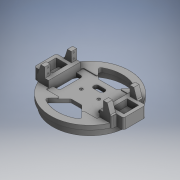
# Autodesk Inventor part: Swivel Top
Saved by Autodesk Inventor 2020.5 (Build 245400000, 400)
## iProperties
Created: 2023-04-01
Part Number: Swivel Top
Material: Generic
Document SubType Name: Modeling
Designer: Wes
Density: 1 g/cm^3
Appearance: Default
Author: Wes
Autodesk Inventor part; units mm, degrees
ref_plane "YZ Plane" through (0, 0, 0) normal (1, 0, 0) x (0, 1, 0)
ref_plane "XZ Plane" through (0, 0, 0) normal (0, 1, 0) x (-1, 0, 0)
ref_plane "XY Plane" through (0, 0, 0) normal (0, 0, 1) x (1, 0, 0)
sketch "Sketch1" plane through (0, 0, 0) normal (0, 0, 1) x (1, 0, 0)
  circle A0 centre (0, 0) radius 74
  dimension "d0" = 148
  constraints: 1 centre point, 1 coincident
  measures "d0" diameter of A0
extrude "Extrusion1" add sketch "Sketch1" along normal blind 8
sketch "Sketch2" plane through (0, 0, 8) normal (0, 0, 1) x (1, 0, 0)
  line L0 (0, 0) -> (0, -55) construction
  line L1 (0, 0) -> (0, 55) construction
  line L2 (0, -55) -> (0, -48) construction
  line L3 (0, -48) -> (-30, -48) construction
  line L4 (0, -48) -> (30, -48) construction
  line L5 (-30, -48) -> (30, -48)
  line L6 (30, -48) -> (30, -71)
  line L7 (30, -71) -> (-30, -71)
  line L8 (-30, -71) -> (-30, -48)
  line L9 (0, -71) -> (0, -84) construction
  line L10 (0, -84) -> (-21, -84) construction
  line L11 (0, -84) -> (21, -84) construction
  line L12 (-21, -84) -> (21, -84)
  line L13 (21, -84) -> (21, -71)
  line L14 (21, -71) -> (-21, -71)
  line L15 (-21, -71) -> (-21, -84)
  dimension "d3" = 55
  dimension "d5" = 7
  dimension "d7" = 30
  dimension "d8" = 60
  dimension "d9" = 23
  dimension "d10" = 13
  dimension "d11" = 21
  dimension "d13" = 42
  dimension "d14" = 13
  dimension "d15" = 60
  constraints: 32 end point, 6 horizontal, 4 parallel, 3 vertical, 2 perpendicular, 1 midpoint, 1 point on line
  measures "d3" distance of L0.start L0.end
  measures "d5" distance of L0.end L2.end
  measures "d7" distance of L2.end L4.end
  measures "d8" distance of L6.end L7.end
  measures "d9" distance of L5.end L6.end
  measures "d10" distance of L9.start L9.end
  measures "d11" distance of L9.end L10.end
  measures "d13" distance of L14.end L13.end
  measures "d14" distance of L13.end L12.end
  measures "d15" distance of L5.end L3.end
extrude "Extrusion2" add sketch "Sketch2" along normal blind 12 and the other way blind 8
sketch "Sketch3" plane through (0, 0, 20) normal (0, 0, 1) x (1, 0, 0)
  line L0 (30, -48) -> (-30, -48) construction
  line L1 (0, -48) -> (0, -55) construction
  line L2 (0, -55) -> (20.2, -55) construction
  line L3 (0, -55) -> (-20.2, -55) construction
  line L4 (20.2, -55) -> (30, -55)
  line L5 (30, -55) -> (30, -62.5)
  line L6 (30, -62.5) -> (20.2, -62.5)
  line L7 (20.2, -62.5) -> (20.2, -55)
  line L8 (-30, -48) -> (-30, -71) projected
  line L9 (-20.2, -55) -> (-30, -55)
  line L10 (-30, -55) -> (-30, -62.5)
  line L11 (-30, -62.5) -> (-20.2, -62.5)
  line L12 (-20.2, -62.5) -> (-20.2, -55)
  point P0 (0, 0)
  dimension "d20" = 7
  dimension "d21" = 20.2
  dimension "d23" = 40.4
  dimension "d24" = 9.8
  dimension "d25" = 7.5
  constraints: 22 end point, 4 horizontal, 4 parallel, 2 perpendicular, 1 midpoint, 1 point on line, 1 vertical
  measures "d20" distance of L1.start L1.end
  measures "d21" distance of L1.end L2.end
  measures "d23" distance of L2.end L3.end
  measures "d24" distance of L5.end L6.end
  measures "d25" distance of L4.end L5.end
extrude "Extrusion3" add sketch "Sketch3" along normal blind 18.5
sketch "Sketch4" plane through (-30, -55, 20) normal (0, 1, 0) x (1, 0, 0)
  line L0 (50.2, -18.5) -> (60, -18.5) construction
  line L1 (54.192715, -18.5) -> (54.192715, -14.845) construction
  line L2 (54.192715, -18.5) -> (57.847715, -18.5) construction
  line L3 (50.2, 0) -> (50.2, -18.5) construction
  line L4 (50.2, -14.845) -> (54.3, -14.845) construction
  line L5 (50.2, -14.845) -> (54.3, -14.845) construction
  circle A0 centre (54.3, -14.845) radius 1.275
  line L6 (54.3, -14.845) -> (54.3, -5.025) construction
  circle A1 centre (54.3, -5.025) radius 1.275
  line L7 (9, 0) -> (51, 0) construction
  line L8 (30, 0) -> (30, -30.194505) construction
  circle A2 centre (5.7, -14.845) radius 1.275
  circle A3 centre (5.7, -5.025) radius 1.275
  point P0 (30, 20)
  dimension "d113" = 18
  dimension "d28" = 3.655
  dimension "d30" = 4.1
  dimension "d32" = 2.55
  dimension "d33" = 9.82
  dimension "d34" = 2.55
  constraints: 12 end point, 4 centre point, 3 horizontal, 3 vertical, 2 coincident, 2 equal length, 2 point on line, 2 symmetric about line, 1 midpoint, 2 other
  measures "d28" distance of L1.start L1.end
  measures "d30" distance of L4.start L4.end
  measures "d32" diameter of A0
  measures "d33" distance of L6.start L6.end
  measures "d34" diameter of A1
extrude "Extrusion4" cut sketch "Sketch4" against normal blind 4.5
mirror "Mirror1" about plane through (0, 0, 0) normal (0, 1, 0) of "Extrusion2", "Extrusion3", "Extrusion4"
sketch "Sketch5" plane through (0, 0, 8) normal (0, 0, 1) x (1, 0, 0)
  line L0 (-30, 0) -> (-35, 0) construction
  line L1 (30, 0) -> (35, 0) construction
  line L2 (-35, -48) -> (35, -48)
  line L3 (35, -48) -> (35, 48)
  line L4 (35, 48) -> (-35, 48)
  line L5 (-35, 48) -> (-35, -48)
  point P0 (0, 0)
  dimension "d37" = 5
  dimension "d38" = 5
  constraints: 12 end point, 3 horizontal, 2 parallel, 1 perpendicular
  measures "d37" distance of L0.start L0.end
  measures "d38" distance of L1.start L1.end
extrude "Extrusion5" cut sketch "Sketch5" against normal blind 1.5
sketch "Sketch6" plane through (0, 0, 0) normal (0, 0, -1) x (-1, 0, 0)
  line L0 (-28.5, -28.5) -> (28.5, -28.5)
  line L1 (28.5, -28.5) -> (28.5, 28.5)
  line L2 (28.5, 28.5) -> (-28.5, 28.5)
  line L3 (-28.5, 28.5) -> (-28.5, -28.5)
  line L4 (-28.5, -28.5) -> (28.5, 28.5) construction
  line L5 (28.5, -28.5) -> (-28.5, 28.5) construction
  line L6 (-36.5, -36.5) -> (36.5, -36.5)
  line L7 (36.5, -36.5) -> (36.5, 36.5)
  line L8 (36.5, 36.5) -> (-36.5, 36.5)
  line L9 (-36.5, 36.5) -> (-36.5, -36.5)
  line L10 (-36.5, -36.5) -> (36.5, 36.5) construction
  line L11 (36.5, -36.5) -> (-36.5, 36.5) construction
  point P0 (0, 0)
  dimension "d41" = 57
  dimension "d42" = 57
  dimension "d43" = 73
  dimension "d44" = 73
  constraints: 24 end point, 4 midpoint, 4 parallel, 2 horizontal, 2 perpendicular
  measures "d41" distance of L2.end L1.end
  measures "d42" distance of L1.end L0.end
  measures "d43" distance of L8.end L7.end
  measures "d44" distance of L7.end L6.end
extrude "Extrusion6" [suppressed]
sketch "Sketch7" plane through (0, 0, 0) normal (0, 0, -1) x (-1, 0, 0)
  line L0 (-28.5, -28.5) -> (28.5, -28.5) construction
  line L1 (-16.505983, -28.5) -> (-16.505983, -20.5) construction
  line L2 (-16.505983, -28.5) -> (-8.505983, -28.5) construction
  line L3 (-28.5, 28.5) -> (-28.5, -28.5) construction
  line L4 (-28.5, -20.5) -> (-20.5, -20.5) construction
  line L5 (-28.5, -20.5) -> (-20.5, -20.5) construction
  circle A0 centre (-20.5, -20.5) radius 1.275
  circle A1 centre (20.5, -20.5) radius 1.275
  circle A2 centre (20.5, 20.5) radius 1.275
  circle A3 centre (-20.5, 20.5) radius 1.275
  point P0 (0, 0)
  dimension "d47" = 8
  dimension "d52" = 8
  dimension "d54" = 2.55
  dimension "d57" = 360
  constraints: 8 end point, 4 centre point, 3 horizontal, 2 equal length, 2 point on line, 1 coincident, 1 vertical, 9 other
  measures "d47" distance of L1.start L1.end
  measures "d52" distance of L4.start L4.end
  measures "d54" diameter of A0
extrude "Extrusion7" [suppressed]
sketch "Sketch8" plane through (0, 0, 0) normal (0, 0, -1) x (-1, 0, 0)
  circle A0 centre (0, 0) radius 70
  circle A1 centre (0, 0) radius 66
  dimension "d61" = 140
  dimension "d62" = 132
  constraints: 2 centre point, 2 coincident
  measures "d61" diameter of A0
  measures "d62" diameter of A1
extrude "Extrusion8" add sketch "Sketch8" along normal blind 12
sketch "Sketch14" plane through (0, 0, 0) normal (0, 0, -1) x (-1, 0, 0)
  circle A0 centre (0, 0) radius 3.15
  dimension "d117" = 6.3
  constraints: 1 centre point
  measures "d117" diameter of A0
extrude "Extrusion13" cut sketch "Sketch14" against normal blind 1.2
sketch "Sketch15" plane through (0, 0, 0) normal (0, 0, -1) x (-1, 0, 0)
  line L0 (-4.392963, -4.05) -> (-6.966247, -6.422385)
  line L1 (4.392963, -4.05) -> (-4.392963, -4.05) construction
  line L2 (-4.392963, -4.05) -> (-4.392963, 4.05) construction
  arc A0 (-4.392963, 4.05) -> (-4.392963, -4.05) centre (0, 0) ccw
  arc A1 (-6.966247, 6.422385) -> (-6.966247, -6.422385) centre (0, 0) ccw
  line L3 (4.392963, -4.05) -> (6.966247, -6.422385)
  line L4 (-4.392963, 4.05) -> (-6.966247, 6.422385)
  line L5 (0, -11.649559) -> (0, 10.698869) construction
  line L6 (4.392963, -4.05) -> (4.392963, 4.05) construction
  circle A2 centre (0, 0) radius 5.975 construction
  arc A3 (4.392963, -4.05) -> (4.392963, 4.05) centre (0, 0) ccw
  arc A4 (6.966247, -6.422385) -> (6.966247, 6.422385) centre (0, 0) ccw
  line L7 (4.392963, 4.05) -> (6.966247, 6.422385)
  point P0 (0, 0)
  point P1 (0, 0)
  point P2 (0, 0)
  dimension "d125" = 11.95
  dimension "d126" = 8.1
  dimension "d127" = 8.1
  dimension "d128" = 3.5
  dimension "d129" = 3.5
  constraints: 16 end point, 12 point on circle, 5 centre point, 2 line through centre, 2 symmetric about line, 2 vertical, 1 concentric, 1 perpendicular, 2 other
  measures "d125" diameter of A2
  measures "d126" distance of L1.start L6.end
  measures "d127" distance of L0.start L2.end
  measures "d128" distance of L0.start L0.end
  measures "d129" distance of L2.end L4.end
extrude "Extrusion14" add sketch "Sketch15" along normal blind 5
sketch "Sketch16" plane through (0, 0, -5) normal (0, 0, -1) x (-1, 0, 0)
  line L0 (4.981142, 4.592259) -> (6.45159, 5.947908)
  line L1 (-4.981142, 4.592259) -> (-6.45159, 5.947908)
  line L2 (-5.975, 0) -> (-6.775, 0) construction
  line L3 (-6.775, 0) -> (-8.775, 0) construction
  arc A0 (-4.981142, 4.592259) -> (-4.981142, -4.592259) centre (0, 0) ccw
  arc A1 (4.981142, -4.592259) -> (4.981142, 4.592259) centre (0, 0) ccw
  circle A2 centre (0, 0) radius 6.775 construction
  arc A3 (-6.45159, 5.947908) -> (-6.45159, -5.947908) centre (0, 0) ccw
  arc A4 (6.45159, -5.947908) -> (6.45159, 5.947908) centre (0, 0) ccw
  line L4 (0, -11.470525) -> (0, 12.047921) construction
  circle A5 centre (0, 0) radius 8.775 construction
  line L5 (6.45159, -5.947908) -> (4.981142, -4.592259)
  line L6 (-6.45159, -5.947908) -> (-4.981142, -4.592259)
  point P0 (-6.231023, 5.744561)
  point P1 (-6.231023, -5.744561)
  dimension "d134" = 0.8
  dimension "d135" = 2
  constraints: 16 point on circle, 14 end point, 6 centre point, 4 symmetric about line, 2 coincident, 2 horizontal, 1 concentric, 1 vertical, 2 other
  measures "d134" distance of L2.start L2.end
  measures "d135" distance of L2.end L3.end
extrude "Extrusion15" add sketch "Sketch16" along normal blind 3.35
sketch "Sketch17" plane through (0, 0, 0) normal (0, 0, -1) x (-1, 0, 0)
  line L0 (0, 0) -> (0, 17.1) construction
  line L1 (0, 0) -> (0, -17.1) construction
  line L2 (0, 0) -> (0, -15.8) construction
  line L3 (0, 0) -> (0, 15.8) construction
  line L4 (0, -15.8) -> (0, -17.1) construction
  line L5 (0, 15.8) -> (0, 17.1) construction
  circle A0 centre (0, 16.45) radius 1.175 construction
  circle A1 centre (0, -16.45) radius 1.175 construction
  circle A2 centre (0, 16.45) radius 1.125
  circle A3 centre (0, -16.45) radius 1.125
  point P0 (0, 0)
  point P1 (0, 0)
  dimension "d138" = 34.2
  dimension "d139" = 31.6
  dimension "d140" = 2.35
  dimension "d141" = 2.35
  dimension "d142" = 2.25
  dimension "d143" = 2.25
  constraints: 12 end point, 4 centre point, 3 coincident, 3 vertical, 2 midpoint, 2 point on line, 1 collinear
  measures "d138" distance of L0.end L1.end
  measures "d139" distance of L3.end L2.end
  measures "d140" diameter of A0
  measures "d141" diameter of A1
  measures "d142" diameter of A2
  measures "d143" diameter of A3
extrude "Extrusion16" cut sketch "Sketch17" against normal up to surface (6.5 mm away)
sketch "Sketch18" plane through (0, 0, 0) normal (0, 0, -1) x (-1, 0, 0)
  line L0 (0, -13.125) -> (-3.125, -13.125) construction
  line L1 (0, -17.625) -> (0, -13.125) construction
  line L2 (0, -16.45) -> (-2.8, -16.45) construction
  line L3 (-2.8, -16.45) -> (-2.605438, -18.440514)
  line L4 (-3.125, -13.125) -> (-2.8, -16.45)
  line L5 (-5.115514, -13.319562) -> (-3.125, -13.125)
  line L6 (-4.790514, -16.644562) -> (-5.115514, -13.319562)
  line L7 (-2.8, -16.45) -> (-4.790514, -16.644562)
  line L8 (-4.595952, -18.635075) -> (-4.790514, -16.644562)
  line L9 (-2.605438, -18.440514) -> (-4.595952, -18.635075)
  line L10 (5.975, 0) -> (-5.975, 0) construction
  line L11 (0, 13.125) -> (-3.125, 13.125) construction
  line L12 (-5.115514, 13.319562) -> (-3.125, 13.125)
  line L13 (0, 16.45) -> (-2.8, 16.45) construction
  line L14 (-3.125, 13.125) -> (-2.8, 16.45)
  line L15 (-2.8, 16.45) -> (-4.790514, 16.644562)
  line L16 (0, 17.625) -> (0, 13.125) construction
  line L17 (-2.8, 16.45) -> (-2.605438, 18.440514)
  line L18 (-2.605438, 18.440514) -> (-4.595952, 18.635075)
  line L19 (-4.595952, 18.635075) -> (-4.790514, 16.644562)
  line L20 (-4.790514, 16.644562) -> (-5.115514, 13.319562)
  line L21 (0, -13.125) -> (3.125, -13.125) construction
  line L22 (0, -16.45) -> (2.8, -16.45) construction
  line L23 (0, -16.45) -> (2.8, -16.45) construction
  line L24 (0, -16.45) -> (2.8, -16.45) construction
  line L25 (2.8, -16.45) -> (2.605438, -18.440514)
  line L26 (2.605438, -18.440514) -> (4.595952, -18.635075)
  line L27 (4.595952, -18.635075) -> (4.790514, -16.644562)
  line L28 (3.125, -13.125) -> (2.8, -16.45)
  line L29 (2.8, -16.45) -> (4.790514, -16.644562)
  line L30 (4.790514, -16.644562) -> (5.115514, -13.319562)
  line L31 (5.115514, -13.319562) -> (3.125, -13.125)
  line L32 (0, 13.125) -> (3.125, 13.125) construction
  line L33 (0, 16.45) -> (2.8, 16.45) construction
  line L34 (0, 16.45) -> (2.8, 16.45) construction
  line L35 (0, 16.45) -> (2.8, 16.45) construction
  line L36 (2.8, 16.45) -> (2.605438, 18.440514)
  line L37 (2.605438, 18.440514) -> (4.595952, 18.635075)
  line L38 (3.125, 13.125) -> (2.8, 16.45)
  line L39 (4.595952, 18.635075) -> (4.790514, 16.644562)
  line L40 (2.8, 16.45) -> (4.790514, 16.644562)
  line L41 (4.790514, 16.644562) -> (5.115514, 13.319562)
  line L42 (5.115514, 13.319562) -> (3.125, 13.125)
  circle A0 centre (0, 16.45) radius 1.125
  line L43 (-4.595952, -18.635075) -> (-5.115514, -13.319562)
  line L44 (-5.115514, -13.319562) -> (-6.110771, -13.416842)
  line L45 (-6.110771, -13.416842) -> (-5.591209, -18.732356)
  line L46 (-5.591209, -18.732356) -> (-4.595952, -18.635075)
  line L47 (4.595952, -18.635075) -> (5.115514, -13.319562)
  line L48 (5.115514, -13.319562) -> (6.110771, -13.416842)
  line L49 (6.110771, -13.416842) -> (5.591209, -18.732356)
  line L50 (5.591209, -18.732356) -> (4.595952, -18.635075)
  line L51 (-5.115514, 13.319562) -> (-4.595952, 18.635075)
  line L52 (-4.595952, 18.635075) -> (-5.591209, 18.732356)
  line L53 (-5.591209, 18.732356) -> (-6.110771, 13.416842)
  line L54 (-6.110771, 13.416842) -> (-5.115514, 13.319562)
  line L55 (5.115514, 13.319562) -> (4.595952, 18.635075)
  line L56 (4.595952, 18.635075) -> (5.591209, 18.732356)
  line L57 (5.591209, 18.732356) -> (6.110771, 13.416842)
  line L58 (6.110771, 13.416842) -> (5.115514, 13.319562)
  point P0 (0, 0)
  point P1 (0, -16.45)
  point P2 (0, -16.45)
  dimension "d146" = 4.5
  dimension "d147" = 6.25
  dimension "d148" = 5.6
  dimension "d149" = 2
  dimension "d150" = 2
  dimension "d153" = 1
  dimension "d154" = 1
  dimension "d155" = 1
  dimension "d156" = 1
  constraints: 118 end point, 22 symmetric about line, 10 perpendicular, 8 parallel, 7 horizontal, 5 collinear, 1 coincident, 1 vertical
  measures "d146" distance of L1.start L0.start
  measures "d147" distance of L0.end L21.end
  measures "d148" distance of L2.end L22.end
  measures "d149" distance of L2.end L8.end
  measures "d150" distance of L2.end L3.end
  measures "d153" distance of L44.end L6.end
  measures "d154" distance of L31.start L48.end
  measures "d155" distance of L52.end L18.end
  measures "d156" distance of L37.end L56.end
extrude "Extrusion17" add sketch "Sketch18" along normal blind 3 contours L7 L6 L5 L4 | L3 L9 L8 L7 | L8 L46 L45 L44 L6 | L20 L15 L14 L12 | L54 L53 L52 L19 L20 | L19 L18 L17 L15 | L29 L27 L26 L25 | L28 L31 L30 L29 | L30 L48 L49 L50 L27 | L40 L41 L42 L38 | L36 L37 L39 L40 | L39 L56 L57 L58 L41
sketch "Sketch19" plane through (0, 0, 6.5) normal (0, 0, 1) x (1, 0, 0)
  circle A0 centre (0, -16.45) radius 1.125 projected
  circle A1 centre (0, -16.45) radius 2.85
  circle A2 centre (0, 16.45) radius 1.125 projected
  circle A3 centre (0, 16.45) radius 2.85
  point P0 (0, 0)
  dimension "d157" = 5.7
  dimension "d158" = 5.7
  constraints: 2 centre point, 2 coincident
  measures "d157" diameter of A1
  measures "d158" diameter of A3
extrude "Extrusion18" cut sketch "Sketch19" against normal blind 1 contours A0 | A1 | A2 | A3
sketch "Sketch10" plane through (0, 0, 20) normal (0, 0, 1) x (1, 0, 0)
  line L0 (21, -84) -> (-21, -84) construction
  line L1 (0, -84) -> (0, -76) construction
  line L2 (35, -48) -> (-35, -48) construction
  line L3 (0, -48) -> (0, -56) construction
  line L4 (0, -48) -> (8, -48) construction
  line L5 (-21, -84) -> (-21, -71) construction
  line L6 (-21, -71) -> (-14, -71) construction
  line L7 (21, -71) -> (21, -84) construction
  line L8 (21, -71) -> (14, -71) construction
  line L9 (-35, -48) -> (-35, 48) construction
  line L10 (-35, 0) -> (35, 0) construction
  line L11 (35, 48) -> (35, -48) construction
  line L12 (-14, -76) -> (14, -76)
  line L13 (14, -76) -> (14, -56)
  line L14 (14, -56) -> (-14, -56)
  line L15 (-14, -56) -> (-14, -76)
  line L16 (-14, 76) -> (14, 76)
  line L17 (14, 76) -> (14, 56)
  line L18 (14, 56) -> (-14, 56)
  line L19 (-14, 56) -> (-14, 76)
  point P0 (0, 0)
  dimension "d70" = 8
  dimension "d71" = 8
  dimension "d73" = 7
  dimension "d74" = 7
  constraints: 28 end point, 4 horizontal, 4 midpoint, 4 symmetric about line, 2 parallel, 2 perpendicular, 2 vertical
  measures "d70" distance of L1.start L1.end
  measures "d71" distance of L3.start L3.end
  measures "d73" distance of L5.end L6.end
  measures "d74" distance of L7.start L8.end
extrude "Extrusion9" cut sketch "Sketch10" against normal blind 12
sketch "Sketch12" plane through (0, 0, 8) normal (0, 0, 1) x (1, 0, 0)
  circle A0 centre (0, 0) radius 3.15
  line L0 (0, 0) -> (34.3, 0) construction
  line L1 (0, 0) -> (-14.3, 0) construction
  line L2 (34.3, 0) -> (34.3, -4.91) construction
  line L3 (34.3, 0) -> (34.3, 4.91) construction
  circle A1 centre (34.3, 4.91) radius 1.5 construction
  circle A2 centre (34.3, -4.91) radius 1.5 construction
  circle A3 centre (-14.3, -4.91) radius 1.5 construction
  circle A4 centre (-14.3, 4.91) radius 1.5 construction
  circle A5 centre (0, 0) radius 66 construction
  line L4 (66, 0) -> (61, 0) construction
  line L5 (-66, 0) -> (-61, 0) construction
  line L6 (29.3, 10) -> (39.3, 10)
  line L7 (39.3, 10) -> (39.3, -10)
  line L8 (39.3, -10) -> (29.3, -10)
  line L9 (29.3, 10) -> (39.3, -10) construction
  line L10 (39.3, 10) -> (29.3, -10) construction
  line L11 (-16.3, 10) -> (-12.3, 10)
  line L12 (-12.3, 10) -> (-12.3, -10)
  line L13 (-16.3, 10) -> (-12.3, -10) construction
  line L14 (-12.3, 10) -> (-16.3, -10) construction
  line L15 (29.3, 10) -> (60.964509, 10) construction
  line L16 (29.3, -10) -> (60.964509, -10) construction
  arc A6 (6.966247, -6.422385) -> (6.966247, 6.422385) centre (0, 0) ccw construction
  line L17 (9.475, 0) -> (25.475, 0) construction
  line L18 (25.475, 10) -> (25.475, -10)
  line L19 (25.475, 10) -> (50.171344, 34.696344)
  line L20 (25.475, 10) -> (60.400904, 10) construction
  line L21 (25.475, -10) -> (50.171344, -34.696344)
  line L22 (25.475, -10) -> (60.400904, -10) construction
  line L23 (-25.475, -10) -> (-25.475, 10)
  line L24 (-25.475, -10) -> (-50.171344, -34.696344)
  line L25 (-25.475, 10) -> (-50.171344, 34.696344)
  line L26 (-30, 48) -> (-30, 55) construction
  line L27 (-30, 48) -> (-22, 48) construction
  line L28 (-35, 48) -> (35, 48) construction
  line L29 (30, 67.646138) -> (30, 48) construction
  line L30 (30, 48) -> (22, 48) construction
  line L31 (-22, 48) -> (22, 48)
  circle A7 centre (0, 16.45) radius 2.85 construction
  line L32 (0, 19.3) -> (0, 35.3) construction
  line L33 (22, 48) -> (22, 35.3)
  line L34 (-22, 48) -> (-22, 35.3)
  line L35 (22, 35.3) -> (-22, 35.3)
  line L36 (22, -48) -> (-22, -48)
  line L37 (22, -48) -> (22, -35.3)
  line L38 (-22, -35.3) -> (22, -35.3)
  line L39 (-22, -48) -> (-22, -35.3)
  arc A8 (-50.171344, 34.696344) -> (-50.171344, -34.696344) centre (0, 0) ccw
  arc A9 (50.171344, -34.696344) -> (-30, 53.113087) centre (0, 0) ccw
  line L40 (-12.3, -10) -> (-22.3, -10)
  line L41 (-12.3, 10) -> (-22.3, 10)
  line L42 (-22.3, 10) -> (-22.3, -10)
  line L43 (-22.3, 0) -> (-32.3, 0) construction
  line L44 (-32.3, 16.825) -> (-32.3, -16.825)
  dimension "d113" = 18
  dimension "d161" = 34.3
  dimension "d162" = 14.3
  dimension "d163" = 4.91
  dimension "d170" = 5
  dimension "d171" = 5
  dimension "d172" = 10
  dimension "d173" = 20
  dimension "d174" = 4
  dimension "d177" = 16
  dimension "d178" = 45
  dimension "d179" = 45
  dimension "d182" = 360
  dimension "d184" = 8
  dimension "d185" = 8
  dimension "d186" = 16
  dimension "d189" = 360
  dimension "d191" = 10
  dimension "d192" = 10
  constraints: 84 end point, 13 horizontal, 9 point on circle, 7 point on line, 7 vertical, 6 centre point, 5 midpoint, 4 coincident, 3 perpendicular, 2 equal length, 1 collinear, 1 parallel, 1 vertical alignment, 33 other
  measures "d161" distance of L0.start L0.end
  measures "d162" distance of L0.start L1.end
  measures "d163" distance of L0.end L2.end
  measures "d170" distance of L4.start L4.end
  measures "d171" distance of L5.start L5.end
  measures "d172" distance of L7.end L8.end
  measures "d173" distance of L6.end L7.end
  measures "d174" distance of L12.end L14.end
  measures "d177" distance of L17.start L17.end
  measures "d178" angle of L20 L19
  measures "d179" angle of L21 L22
  measures "d184" distance of L26.start L27.end
  measures "d185" distance of L29.end L30.end
  measures "d186" distance of L32.start L32.end
  measures "d191" distance of L12.end L40.end
  measures "d192" distance of L43.start L43.end
extrude "Extrusion11" cut sketch "Sketch12" against normal up to surface (8 mm away) contours L11 L12 L40 L42 L41 | L19 A9 L21 L18 | L24 A8 L25 L44 | L31 L33 L35 L34 | L36 L39 L38 L37
sketch "Sketch20" plane through (0, 0, 8) normal (0, 0, 1) x (1, 0, 0)
  circle A0 centre (0, 0) radius 74
  line L0 (-14, 56) -> (-14, 76)
  line L1 (-14, 72.663608) -> (-14, 77.663608)
  line L2 (-14, 77.663608) -> (14, 77.663608)
  line L3 (14, 76) -> (14, 56)
  line L4 (14, 77.663608) -> (14, 72.663608)
  line L5 (14, -72.663608) -> (14, -77.663608)
  line L6 (14, -77.663608) -> (-14, -77.663608)
  line L7 (-14, -77.663608) -> (-14, -72.663608)
  dimension "d195" = 5
  dimension "d198" = 360
  constraints: 12 end point, 2 point on circle, 2 point on line, 1 centre point, 1 coincident, 1 collinear, 1 perpendicular, 15 other
  measures "d195" distance of L1.start L1.end
extrude "Extrusion19" cut sketch "Sketch20" along normal blind 12 and the other way blind 8 contours A0 L0 L1 L2 L4 L3 | L5 L6 L7 A0
sketch "Sketch13" plane through (0, 0, 8) normal (0, 0, 1) x (1, 0, 0)
  line L0 (-36.5, 29.5) -> (-36.5, -29.5)
  line L1 (-35, -48) -> (-35, 48)
  line L2 (-36.5, -29.5) -> (-53.392415, -29.5)
  line L3 (-35, 29.5) -> (-36.5, 29.5)
  line L4 (-36.5, 29.5) -> (-36.5, -29.5)
  line L5 (-36.5, -29.5) -> (-35, -29.5)
  line L6 (-35, -29.5) -> (-35, 29.5)
  line L7 (35, 48) -> (35, -48)
  line L8 (36.5, -29.5) -> (36.5, 29.5)
  line L9 (35, -29.5) -> (36.5, -29.5)
  line L10 (36.5, -29.5) -> (36.5, 29.5)
  line L11 (36.5, 29.5) -> (35, 29.5)
  line L12 (35, 29.5) -> (35, -29.5)
  point P0 (0, 0)
  constraints: 16 end point, 4 parallel, 2 horizontal, 2 perpendicular, 2 point on line
extrude "Extrusion12" [suppressed]
draft "FaceDraft1" angle 18 pull direction (0, 0, 1) faces at (-26.733333, -62.5, 26.166667) (23.466667, -62.5, 26.166667) (-26.733333, 62.5, 26.166667) (23.466667, 62.5, 26.166667) fixed edges at (-25.1, -62.5, 38.5) (25.1, -62.5, 38.5) (-25.1, 62.5, 38.5) (25.1, 62.5, 38.5)
fillet "Fillet1" radius 4 24 edges at (21, -84, 10) (-21, -84, 10) (21, 84, 10) (-21, 84, 10) (30, 71, 10) (-30, 71, 10) (30, -71, 10) (-30, -71, 10) (-50.1713, -34.6963, 4) (-50.1713, 34.6963, 4) (22, 35.3, 3.25) (-22, 35.3, 3.25) (-22, -35.3, 3.25) (22, -35.3, 3.25) (25.475, -10, 3.25) (25.475, 10, 3.25) (-32.3, 16.825, 3.25) (-32.3, -16.825, 3.25) (50.1713, 34.6963, 4) (50.1713, -34.6963, 4) (-22.3, -10, 3.25) (-12.3, -10, 3.25) (-22.3, 10, 3.25) (-12.3, 10, 3.25)
fillet "Fillet2" radius 2 4 edges at (-24.9518, -68.511, 20) (24.9518, -68.511, 20) (24.9518, 68.511, 20) (-24.9518, 68.511, 20)
fillet "Fillet4" radius 2 8 edges at (-35, -19.525, 7.25) (-35, 19.525, 7.25) (35, 19.525, 7.25) (35, -19.525, 7.25) (-35, -48, 7.25) (35, -48, 7.25) (-35, 48, 7.25) (35, 48, 7.25)
fillet "Fillet5" radius 3 10 edges at (-5.851, -16.0746, 0) (5.851, 16.0746, 0) (-5.851, 16.0746, 0) (5.851, -16.0746, 0) (6.775, 0, -5) (-6.775, 0, -5) (-8.775, 0, -5) (-9.475, 0, 0) (8.775, 0, -5) (9.475, 0, 0)
body "Solid1"
